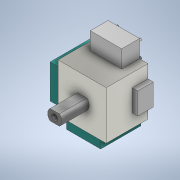
# Autodesk Inventor part: Joystick
Saved by Autodesk Inventor 2020 (Build 240168000, 168)
## iProperties
Created: 2021-01-14
Part Number: Joystick
Material: Generic
Document SubType Name: Modeling
Designer: Luke
Density: 1 g/cm^3
Appearance: Default
Author: Luke
Autodesk Inventor part; units mm, degrees
ref_plane "YZ Plane" through (0, 0, 0) normal (1, 0, 0) x (0, 1, 0)
ref_plane "XZ Plane" through (0, 0, 0) normal (0, 1, 0) x (-1, 0, 0)
ref_plane "XY Plane" through (0, 0, 0) normal (0, 0, 1) x (1, 0, 0)
sketch "Sketch1" plane through (0, 0, 0) normal (0, 0, 1) x (1, 0, 0)
  line L0 (-6.6921, -30.344) -> (6.8079, -30.344)
  line L1 (6.8079, -30.344) -> (6.8079, -43.844)
  line L2 (6.8079, -43.844) -> (-6.6921, -43.844)
  line L3 (-6.6921, -43.844) -> (-6.6921, -30.344)
  line L4 (-6.6921, -30.344) -> (6.8079, -43.844) construction
  line L5 (6.8079, -30.344) -> (-6.6921, -43.844) construction
  line L6 (-4.7071, -46.444) -> (4.8229, -46.444)
  line L7 (4.8229, -46.444) -> (4.8229, -43.844)
  line L8 (4.8229, -43.844) -> (-4.7071, -43.844)
  line L9 (-4.7071, -43.844) -> (-4.7071, -46.444)
  line L10 (-9.2921, -32.329) -> (-6.6921, -32.329)
  line L11 (-6.6921, -32.329) -> (-6.6921, -41.859)
  line L12 (-6.6921, -41.859) -> (-9.2921, -41.859)
  line L13 (-9.2921, -41.859) -> (-9.2921, -32.329)
  line L14 (6.8079, -34.044) -> (8.3079, -34.044)
  line L15 (8.3079, -34.044) -> (8.3079, -40.144)
  line L16 (8.3079, -40.144) -> (6.8079, -40.144)
  line L17 (6.8079, -40.144) -> (6.8079, -34.044)
  point P0 (0, 0)
  point P1 (0.0579, -37.094)
  point P2 (0.0579, -43.844)
  point P3 (-6.6921, -37.094)
  point P4 (-6.6921, -37.094)
  point P5 (-9.2921, -37.094)
  point P6 (6.8079, -37.094)
  point P7 (8.3079, -37.094)
  point P8 (8.3079, -37.094)
  point P9 (6.8079, -37.094)
  dimension "d0" = 13.5
  dimension "d1" = 13.5
  dimension "d3" = 9.53
  dimension "d4" = 2.6
  dimension "d7" = 2.6
  dimension "d8" = 9.53
  dimension "d19" = 1.5
  dimension "d20" = 6.1
  constraints: 36 end point, 8 parallel, 7 midpoint, 4 horizontal, 4 perpendicular
  measures "d0" distance of L1.end L2.end
  measures "d1" distance of L0.end L1.end
  measures "d3" distance of L8.end L7.end
  measures "d4" distance of L7.end L6.end
  measures "d7" distance of L11.end L12.end
  measures "d8" distance of L10.end L11.end
  measures "d19" distance of L15.end L16.end
  measures "d20" distance of L14.end L15.end
extrude "Extrusion1" add sketch "Sketch1" along normal blind 11.69 contours L0 L1 L2 L3
ref_plane "Work Plane2" through (0, 0, 0) normal (0, 0, 1) x (1, 0, 0)
ref_plane "Work Plane3" through (0, 0, 0) normal (0, 0, 1) x (1, 0, 0)
sketch "Sketch3" plane through (0, 0, 0) normal (0, 0, 1) x (1, 0, 0)
  line L0 (-6.6921, -30.344) -> (6.8079, -30.344)
  line L1 (6.8079, -30.344) -> (6.8079, -43.844)
  line L2 (6.8079, -43.844) -> (-6.6921, -43.844)
  line L3 (-6.6921, -43.844) -> (-6.6921, -30.344)
  line L4 (-6.6921, -30.344) -> (6.8079, -43.844) construction
  line L5 (6.8079, -30.344) -> (-6.6921, -43.844) construction
  line L6 (-4.7071, -46.444) -> (4.8229, -46.444)
  line L7 (4.8229, -46.444) -> (4.8229, -43.844)
  line L8 (4.8229, -43.844) -> (-4.7071, -43.844)
  line L9 (-4.7071, -43.844) -> (-4.7071, -46.444)
  line L10 (-9.2921, -32.329) -> (-6.6921, -32.329)
  line L11 (-6.6921, -32.329) -> (-6.6921, -41.859)
  line L12 (-6.6921, -41.859) -> (-9.2921, -41.859)
  line L13 (-9.2921, -41.859) -> (-9.2921, -32.329)
  line L14 (6.8079, -34.044) -> (8.3079, -34.044)
  line L15 (8.3079, -34.044) -> (8.3079, -40.144)
  line L16 (8.3079, -40.144) -> (6.8079, -40.144)
  line L17 (6.8079, -40.144) -> (6.8079, -34.044)
  point P0 (0, 0)
  point P1 (0, 0)
  point P2 (0.0579, -37.094)
  point P3 (0.0579, -43.844)
  point P4 (-6.6921, -37.094)
  point P5 (-6.6921, -37.094)
  point P6 (-9.2921, -37.094)
  point P7 (6.8079, -37.094)
  point P8 (6.8079, -37.094)
  point P9 (8.3079, -37.094)
  point P10 (8.3079, -37.094)
  dimension "d21" = 13.5
  dimension "d22" = 13.5
  dimension "d23" = 9.53
  dimension "d24" = 2.6
  dimension "d25" = 2.6
  dimension "d26" = 9.53
  dimension "d27" = 1.5
  dimension "d28" = 6.1
  constraints: 36 end point, 8 parallel, 7 midpoint, 4 horizontal, 4 perpendicular
  measures "d21" distance of L1.end L2.end
  measures "d22" distance of L0.end L1.end
  measures "d23" distance of L8.end L7.end
  measures "d24" distance of L7.end L6.end
  measures "d25" distance of L11.end L12.end
  measures "d26" distance of L10.end L11.end
  measures "d27" distance of L15.end L16.end
  measures "d28" distance of L14.end L15.end
extrude "Extrusion2" add sketch "Sketch3" along normal blind 11.27 contours L3 L12 L13 L10 | L2 L7 L6 L9
ref_plane "Work Plane4" through (0, 0, 0) normal (0, 0, 1) x (1, 0, 0)
sketch "Sketch4" plane through (0, 0, 0) normal (0, 0, 1) x (1, 0, 0)
  line L0 (-6.6921, -30.344) -> (6.8079, -30.344)
  line L1 (6.8079, -30.344) -> (6.8079, -43.844)
  line L2 (6.8079, -43.844) -> (-6.6921, -43.844)
  line L3 (-6.6921, -43.844) -> (-6.6921, -30.344)
  line L4 (-6.6921, -30.344) -> (6.8079, -43.844) construction
  line L5 (6.8079, -30.344) -> (-6.6921, -43.844) construction
  line L6 (-4.7071, -46.444) -> (4.8229, -46.444)
  line L7 (4.8229, -46.444) -> (4.8229, -43.844)
  line L8 (4.8229, -43.844) -> (-4.7071, -43.844)
  line L9 (-4.7071, -43.844) -> (-4.7071, -46.444)
  line L10 (-9.2921, -32.329) -> (-6.6921, -32.329)
  line L11 (-6.6921, -32.329) -> (-6.6921, -41.859)
  line L12 (-6.6921, -41.859) -> (-9.2921, -41.859)
  line L13 (-9.2921, -41.859) -> (-9.2921, -32.329)
  line L14 (6.8079, -34.044) -> (8.3079, -34.044)
  line L15 (8.3079, -34.044) -> (8.3079, -40.144)
  line L16 (8.3079, -40.144) -> (6.8079, -40.144)
  line L17 (6.8079, -40.144) -> (6.8079, -34.044)
  point P0 (0, 0)
  point P1 (0, 0)
  point P2 (0, 0)
  point P3 (6.8079, -37.094)
  point P4 (0.0579, -43.844)
  point P5 (-6.6921, -37.094)
  point P6 (0.0579, -37.094)
  point P7 (-6.6921, -37.094)
  point P8 (-9.2921, -37.094)
  point P9 (8.3079, -37.094)
  point P10 (6.8079, -37.094)
  point P11 (8.3079, -37.094)
  dimension "d31" = 13.5
  dimension "d32" = 13.5
  dimension "d33" = 9.53
  dimension "d34" = 2.6
  dimension "d35" = 2.6
  dimension "d36" = 9.53
  dimension "d37" = 1.5
  dimension "d38" = 6.1
  constraints: 36 end point, 8 parallel, 7 midpoint, 4 horizontal, 4 perpendicular
  measures "d31" distance of L1.end L2.end
  measures "d32" distance of L0.end L1.end
  measures "d33" distance of L8.end L7.end
  measures "d34" distance of L7.end L6.end
  measures "d35" distance of L11.end L12.end
  measures "d36" distance of L10.end L11.end
  measures "d37" distance of L15.end L16.end
  measures "d38" distance of L14.end L15.end
extrude "Extrusion3" add sketch "Sketch4" along normal blind 4.38 contours L14 L15 L16 L1
sketch "Sketch5" plane through (0, 0, 11.69) normal (0, 0, 1) x (1, 0, 0)
  line L0 (-6.6921, -30.344) -> (-6.6921, -43.844) projected
  line L1 (-6.6921, -43.844) -> (6.8079, -43.844) projected
  line L2 (6.8079, -43.844) -> (6.8079, -30.344) projected
  line L3 (6.8079, -30.344) -> (-6.6921, -30.344) projected
  line L4 (6.8079, -30.344) -> (-6.6921, -30.344) projected
  line L5 (6.8079, -43.844) -> (6.8079, -40.144) projected
  line L6 (-6.6921, -30.344) -> (-6.6921, -32.329) projected
  line L7 (1.3808, -38.594) -> (-1.2649, -38.594)
  line L8 (-1.2649, -35.594) -> (1.3808, -35.594)
  arc A0 (1.3808, -38.594) -> (1.3808, -35.594) centre (0.0579, -37.094) ccw
  arc A1 (-1.2649, -35.594) -> (-1.2649, -38.594) centre (0.0579, -37.094) ccw
  circle A2 centre (0.0579, -37.094) radius 0.845
  point P0 (0, 0)
  dimension "d44" = 1.69
  constraints: 4 end point, 4 point on circle, 3 centre point, 2 coincident, 1 horizontal, 1 parallel
  measures "d44" diameter of A2
extrude "Extrusion4" add sketch "Sketch5" along normal blind 7.67 contours L7 A1 L8 A0
sketch "Sketch6" plane through (0, 0, 0) normal (0, 0, -1) x (-1, 0, 0)
  circle A0 centre (2.4821, -45.984) radius 0.3395 projected
  circle A1 centre (8.832, -39.634) radius 0.3395 projected
  circle A2 centre (8.832, -37.094) radius 0.3395 projected
  circle A3 centre (8.832, -34.554) radius 0.3395 projected
  circle A4 centre (-0.0579, -45.984) radius 0.3395 projected
  circle A5 centre (-2.5979, -45.984) radius 0.3395 projected
  circle A6 centre (-3.2329, -31.4425) radius 0.3395 projected
  circle A7 centre (-3.2329, -26.9975) radius 0.3395 projected
  circle A8 centre (3.117, -31.4425) radius 0.3395 projected
  circle A9 centre (3.1171, -26.9975) radius 0.3395 projected
  point P0 (0, 0)
extrude "Extrusion5" add sketch "Sketch6" along normal blind 1.5
sketch "Sketch7" plane through (0, 0, 0) normal (0, 0, -1) x (-1, 0, 0)
  line L0 (-4.4579, -30.344) -> (4.3421, -30.344)
  line L1 (4.3421, -30.344) -> (4.3421, -25.424)
  line L2 (4.3421, -25.424) -> (-4.4579, -25.424)
  line L3 (-4.4579, -25.424) -> (-4.4579, -30.344)
  line L4 (-6.8079, -30.344) -> (6.6921, -30.344) projected
  point P0 (0, 0)
  point P1 (-0.0579, -30.344)
  point P2 (-0.0579, -30.344)
  dimension "d49" = 8.8
  dimension "d50" = 4.92
  constraints: 8 end point, 2 midpoint, 2 parallel, 1 horizontal, 1 perpendicular
  measures "d49" distance of L2.end L1.end
  measures "d50" distance of L1.end L0.end
extrude "Extrusion6" add sketch "Sketch7" against normal blind 5
body "Solid1"
